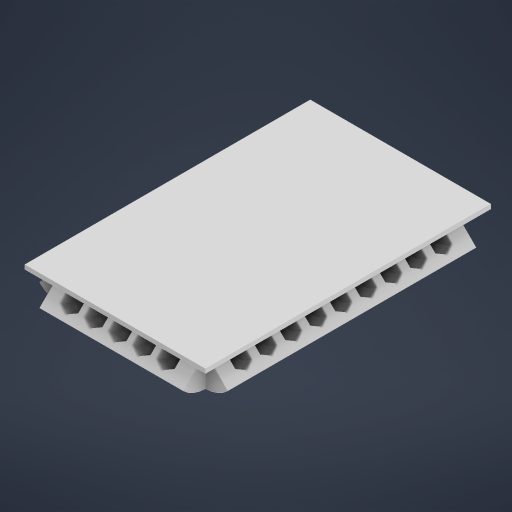
# Autodesk Inventor part: cap
Saved by Autodesk Inventor 2023 (Build 270158000, 158)
## iProperties
Created: 2022-02-14
Part Number: cap
Material: Generic
Document SubType Name: Modeling
Designer: Vlasciar
Density: 1 g/cm^3
Appearance: Default
Author: Vlasciar
Autodesk Inventor part; units mm, degrees
ref_plane "YZ Plane" through (0, 0, 0) normal (1, 0, 0) x (0, 1, 0)
ref_plane "XZ Plane" through (0, 0, 0) normal (0, 1, 0) x (-1, 0, 0)
ref_plane "XY Plane" through (0, 0, 0) normal (0, 0, 1) x (1, 0, 0)
sketch "Sketch1" plane through (0, 0, 0) normal (0, 1, 0) x (-1, 0, 0)
  line L0 (45.3593, 21.0458) -> (-32.1407, 21.0458)
  line L1 (-32.1407, 21.0458) -> (-32.1407, -112.9542)
  line L2 (-32.1407, -112.9542) -> (45.3593, -112.9542)
  line L3 (45.3593, -112.9542) -> (45.3593, 21.0458)
  line L4 (50.3593, 26.0458) -> (-37.1407, 26.0458)
  line L5 (-37.1407, 26.0458) -> (-37.1407, -117.9542)
  line L6 (-37.1407, -117.9542) -> (50.3593, -117.9542)
  line L7 (50.3593, -117.9542) -> (50.3593, 26.0458)
  point P0 (0, 0)
  dimension "d0" = 77.5
  dimension "d1" = 134
  dimension "d2" = 5
  dimension "d3" = 5
  dimension "d4" = 5
  dimension "d5" = 5
  constraints: 16 end point, 4 parallel, 2 horizontal, 2 perpendicular
  measures "d0" distance of L0.start L0.end
  measures "d1" distance of L2.end L0.start
  measures "d2" distance between parallel lines of L7 L3
  measures "d3" distance between parallel lines of L0 L4
  measures "d4" distance between parallel lines of L1 L5
  measures "d5" distance between parallel lines of L6 L2
extrude "Extrusion1" add sketch "Sketch1" against normal blind 3 contours L3 L2 L1 L0
extrude "Extrusion2" add sketch "Sketch1" along normal blind 2 contours L3 L2 L1 L0 | L7 L6 L5 L4
shell "Shell1" thickness 4 removed faces 1 at (-19.526, -3, -68.2876)
sketch "Sketch2" plane through (-41.3593, -2, 17.0458) normal (0, -1, 0) x (1, 0, 0)
  line L0 (69.5, 0) -> (69.5, -126) projected
  line L1 (0, 0) -> (69.5, 0) projected
  line L2 (0, -126) -> (0, 0) projected
  line L3 (69.5, -126) -> (0, -126) projected
  point P0 (41.3593, -17.0458)
extrude "Extrusion3" cut sketch "Sketch2" against normal blind 1
sketch "Sketch3" plane through (-41.3593, -1, 17.0458) normal (0, -1, 0) x (1, 0, 0)
  line L0 (69.5, 0) -> (69.5, -126) projected
  line L1 (0, 0) -> (69.5, 0) projected
  line L2 (60.5, -10.9282) -> (60.5, -6.3094)
  line L3 (60.5, -6.3094) -> (64.5, -4)
  line L4 (64.5, -4) -> (68.5, -6.3094)
  line L5 (68.5, -6.3094) -> (68.5, -10.9282)
  line L6 (68.5, -10.9282) -> (64.5, -13.2376)
  line L7 (64.5, -13.2376) -> (60.5, -10.9282)
  line L8 (69.5, 0) -> (69.5, -126) projected
  line L9 (0, -126) -> (0, 0) projected
  line L10 (60.5, -22.9282) -> (60.5, -18.3094)
  line L11 (60.5, -18.3094) -> (64.5, -16)
  line L12 (64.5, -16) -> (68.5, -18.3094)
  line L13 (68.5, -18.3094) -> (68.5, -22.9282)
  line L14 (68.5, -22.9282) -> (64.5, -25.2376)
  line L15 (64.5, -25.2376) -> (60.5, -22.9282)
  line L16 (60.5, -34.9282) -> (60.5, -30.3094)
  line L17 (60.5, -30.3094) -> (64.5, -28)
  line L18 (64.5, -28) -> (68.5, -30.3094)
  line L19 (68.5, -30.3094) -> (68.5, -34.9282)
  line L20 (68.5, -34.9282) -> (64.5, -37.2376)
  line L21 (64.5, -37.2376) -> (60.5, -34.9282)
  line L22 (60.5, -46.9282) -> (60.5, -42.3094)
  line L23 (60.5, -42.3094) -> (64.5, -40)
  line L24 (64.5, -40) -> (68.5, -42.3094)
  line L25 (68.5, -42.3094) -> (68.5, -46.9282)
  line L26 (68.5, -46.9282) -> (64.5, -49.2376)
  line L27 (64.5, -49.2376) -> (60.5, -46.9282)
  line L28 (60.5, -58.9282) -> (60.5, -54.3094)
  line L29 (60.5, -54.3094) -> (64.5, -52)
  line L30 (64.5, -52) -> (68.5, -54.3094)
  line L31 (68.5, -54.3094) -> (68.5, -58.9282)
  line L32 (68.5, -58.9282) -> (64.5, -61.2376)
  line L33 (64.5, -61.2376) -> (60.5, -58.9282)
  line L34 (60.5, -70.9282) -> (60.5, -66.3094)
  line L35 (60.5, -66.3094) -> (64.5, -64)
  line L36 (64.5, -64) -> (68.5, -66.3094)
  line L37 (68.5, -66.3094) -> (68.5, -70.9282)
  line L38 (68.5, -70.9282) -> (64.5, -73.2376)
  line L39 (64.5, -73.2376) -> (60.5, -70.9282)
  line L40 (60.5, -82.9282) -> (60.5, -78.3094)
  line L41 (60.5, -78.3094) -> (64.5, -76)
  line L42 (64.5, -76) -> (68.5, -78.3094)
  line L43 (68.5, -78.3094) -> (68.5, -82.9282)
  line L44 (68.5, -82.9282) -> (64.5, -85.2376)
  line L45 (64.5, -85.2376) -> (60.5, -82.9282)
  line L46 (60.5, -94.9282) -> (60.5, -90.3094)
  line L47 (60.5, -90.3094) -> (64.5, -88)
  line L48 (64.5, -88) -> (68.5, -90.3094)
  line L49 (68.5, -90.3094) -> (68.5, -94.9282)
  line L50 (68.5, -94.9282) -> (64.5, -97.2376)
  line L51 (64.5, -97.2376) -> (60.5, -94.9282)
  line L52 (60.5, -106.9282) -> (60.5, -102.3094)
  line L53 (60.5, -102.3094) -> (64.5, -100)
  line L54 (64.5, -100) -> (68.5, -102.3094)
  line L55 (68.5, -102.3094) -> (68.5, -106.9282)
  line L56 (68.5, -106.9282) -> (64.5, -109.2376)
  line L57 (64.5, -109.2376) -> (60.5, -106.9282)
  line L58 (60.5, -118.9282) -> (60.5, -114.3094)
  line L59 (60.5, -114.3094) -> (64.5, -112)
  line L60 (64.5, -112) -> (68.5, -114.3094)
  line L61 (68.5, -114.3094) -> (68.5, -118.9282)
  line L62 (68.5, -118.9282) -> (64.5, -121.2376)
  line L63 (64.5, -121.2376) -> (60.5, -118.9282)
  line L64 (48.5, -10.9282) -> (48.5, -6.3094)
  line L65 (48.5, -6.3094) -> (52.5, -4)
  line L66 (52.5, -4) -> (56.5, -6.3094)
  line L67 (56.5, -6.3094) -> (56.5, -10.9282)
  line L68 (56.5, -10.9282) -> (52.5, -13.2376)
  line L69 (52.5, -13.2376) -> (48.5, -10.9282)
  line L70 (48.5, -22.9282) -> (48.5, -18.3094)
  line L71 (48.5, -18.3094) -> (52.5, -16)
  line L72 (52.5, -16) -> (56.5, -18.3094)
  line L73 (56.5, -18.3094) -> (56.5, -22.9282)
  line L74 (56.5, -22.9282) -> (52.5, -25.2376)
  line L75 (52.5, -25.2376) -> (48.5, -22.9282)
  line L76 (48.5, -34.9282) -> (48.5, -30.3094)
  line L77 (48.5, -30.3094) -> (52.5, -28)
  line L78 (52.5, -28) -> (56.5, -30.3094)
  line L79 (56.5, -30.3094) -> (56.5, -34.9282)
  line L80 (56.5, -34.9282) -> (52.5, -37.2376)
  line L81 (52.5, -37.2376) -> (48.5, -34.9282)
  line L82 (48.5, -46.9282) -> (48.5, -42.3094)
  line L83 (48.5, -42.3094) -> (52.5, -40)
  line L84 (52.5, -40) -> (56.5, -42.3094)
  line L85 (56.5, -42.3094) -> (56.5, -46.9282)
  line L86 (56.5, -46.9282) -> (52.5, -49.2376)
  line L87 (52.5, -49.2376) -> (48.5, -46.9282)
  line L88 (48.5, -58.9282) -> (48.5, -54.3094)
  line L89 (48.5, -54.3094) -> (52.5, -52)
  line L90 (52.5, -52) -> (56.5, -54.3094)
  line L91 (56.5, -54.3094) -> (56.5, -58.9282)
  line L92 (56.5, -58.9282) -> (52.5, -61.2376)
  line L93 (52.5, -61.2376) -> (48.5, -58.9282)
  line L94 (48.5, -70.9282) -> (48.5, -66.3094)
  line L95 (48.5, -66.3094) -> (52.5, -64)
  line L96 (52.5, -64) -> (56.5, -66.3094)
  line L97 (56.5, -66.3094) -> (56.5, -70.9282)
  line L98 (56.5, -70.9282) -> (52.5, -73.2376)
  line L99 (52.5, -73.2376) -> (48.5, -70.9282)
  line L100 (48.5, -82.9282) -> (48.5, -78.3094)
  line L101 (48.5, -78.3094) -> (52.5, -76)
  line L102 (52.5, -76) -> (56.5, -78.3094)
  line L103 (56.5, -78.3094) -> (56.5, -82.9282)
  line L104 (56.5, -82.9282) -> (52.5, -85.2376)
  line L105 (52.5, -85.2376) -> (48.5, -82.9282)
  line L106 (48.5, -94.9282) -> (48.5, -90.3094)
  line L107 (48.5, -90.3094) -> (52.5, -88)
  line L108 (52.5, -88) -> (56.5, -90.3094)
  line L109 (56.5, -90.3094) -> (56.5, -94.9282)
  line L110 (56.5, -94.9282) -> (52.5, -97.2376)
  line L111 (52.5, -97.2376) -> (48.5, -94.9282)
  line L112 (48.5, -106.9282) -> (48.5, -102.3094)
  line L113 (48.5, -102.3094) -> (52.5, -100)
  line L114 (52.5, -100) -> (56.5, -102.3094)
  line L115 (56.5, -102.3094) -> (56.5, -106.9282)
  line L116 (56.5, -106.9282) -> (52.5, -109.2376)
  line L117 (52.5, -109.2376) -> (48.5, -106.9282)
  line L118 (48.5, -118.9282) -> (48.5, -114.3094)
  line L119 (48.5, -114.3094) -> (52.5, -112)
  line L120 (52.5, -112) -> (56.5, -114.3094)
  line L121 (56.5, -114.3094) -> (56.5, -118.9282)
  line L122 (56.5, -118.9282) -> (52.5, -121.2376)
  line L123 (52.5, -121.2376) -> (48.5, -118.9282)
  line L124 (36.5, -10.9282) -> (36.5, -6.3094)
  line L125 (36.5, -6.3094) -> (40.5, -4)
  line L126 (40.5, -4) -> (44.5, -6.3094)
  line L127 (44.5, -6.3094) -> (44.5, -10.9282)
  line L128 (44.5, -10.9282) -> (40.5, -13.2376)
  line L129 (40.5, -13.2376) -> (36.5, -10.9282)
  line L130 (36.5, -22.9282) -> (36.5, -18.3094)
  line L131 (36.5, -18.3094) -> (40.5, -16)
  line L132 (40.5, -16) -> (44.5, -18.3094)
  line L133 (44.5, -18.3094) -> (44.5, -22.9282)
  line L134 (44.5, -22.9282) -> (40.5, -25.2376)
  line L135 (40.5, -25.2376) -> (36.5, -22.9282)
  line L136 (36.5, -34.9282) -> (36.5, -30.3094)
  line L137 (36.5, -30.3094) -> (40.5, -28)
  line L138 (40.5, -28) -> (44.5, -30.3094)
  line L139 (44.5, -30.3094) -> (44.5, -34.9282)
  line L140 (44.5, -34.9282) -> (40.5, -37.2376)
  line L141 (40.5, -37.2376) -> (36.5, -34.9282)
  line L142 (36.5, -46.9282) -> (36.5, -42.3094)
  line L143 (36.5, -42.3094) -> (40.5, -40)
  line L144 (40.5, -40) -> (44.5, -42.3094)
  line L145 (44.5, -42.3094) -> (44.5, -46.9282)
  line L146 (44.5, -46.9282) -> (40.5, -49.2376)
  line L147 (40.5, -49.2376) -> (36.5, -46.9282)
  line L148 (36.5, -58.9282) -> (36.5, -54.3094)
  line L149 (36.5, -54.3094) -> (40.5, -52)
  line L150 (40.5, -52) -> (44.5, -54.3094)
  line L151 (44.5, -54.3094) -> (44.5, -58.9282)
  line L152 (44.5, -58.9282) -> (40.5, -61.2376)
  line L153 (40.5, -61.2376) -> (36.5, -58.9282)
  line L154 (36.5, -70.9282) -> (36.5, -66.3094)
  line L155 (36.5, -66.3094) -> (40.5, -64)
  line L156 (40.5, -64) -> (44.5, -66.3094)
  line L157 (44.5, -66.3094) -> (44.5, -70.9282)
  line L158 (44.5, -70.9282) -> (40.5, -73.2376)
  line L159 (40.5, -73.2376) -> (36.5, -70.9282)
  line L160 (36.5, -82.9282) -> (36.5, -78.3094)
  line L161 (36.5, -78.3094) -> (40.5, -76)
  line L162 (40.5, -76) -> (44.5, -78.3094)
  line L163 (44.5, -78.3094) -> (44.5, -82.9282)
  line L164 (44.5, -82.9282) -> (40.5, -85.2376)
  line L165 (40.5, -85.2376) -> (36.5, -82.9282)
  line L166 (36.5, -94.9282) -> (36.5, -90.3094)
  line L167 (36.5, -90.3094) -> (40.5, -88)
  line L168 (40.5, -88) -> (44.5, -90.3094)
  line L169 (44.5, -90.3094) -> (44.5, -94.9282)
  line L170 (44.5, -94.9282) -> (40.5, -97.2376)
  line L171 (40.5, -97.2376) -> (36.5, -94.9282)
  line L172 (36.5, -106.9282) -> (36.5, -102.3094)
  line L173 (36.5, -102.3094) -> (40.5, -100)
  line L174 (40.5, -100) -> (44.5, -102.3094)
  line L175 (44.5, -102.3094) -> (44.5, -106.9282)
  line L176 (44.5, -106.9282) -> (40.5, -109.2376)
  line L177 (40.5, -109.2376) -> (36.5, -106.9282)
  line L178 (36.5, -118.9282) -> (36.5, -114.3094)
  line L179 (36.5, -114.3094) -> (40.5, -112)
  line L180 (40.5, -112) -> (44.5, -114.3094)
  line L181 (44.5, -114.3094) -> (44.5, -118.9282)
  line L182 (44.5, -118.9282) -> (40.5, -121.2376)
  line L183 (40.5, -121.2376) -> (36.5, -118.9282)
  line L184 (24.5, -10.9282) -> (24.5, -6.3094)
  line L185 (24.5, -6.3094) -> (28.5, -4)
  line L186 (28.5, -4) -> (32.5, -6.3094)
  line L187 (32.5, -6.3094) -> (32.5, -10.9282)
  line L188 (32.5, -10.9282) -> (28.5, -13.2376)
  line L189 (28.5, -13.2376) -> (24.5, -10.9282)
  line L190 (24.5, -22.9282) -> (24.5, -18.3094)
  line L191 (24.5, -18.3094) -> (28.5, -16)
  line L192 (28.5, -16) -> (32.5, -18.3094)
  line L193 (32.5, -18.3094) -> (32.5, -22.9282)
  line L194 (32.5, -22.9282) -> (28.5, -25.2376)
  line L195 (28.5, -25.2376) -> (24.5, -22.9282)
  line L196 (24.5, -34.9282) -> (24.5, -30.3094)
  line L197 (24.5, -30.3094) -> (28.5, -28)
  line L198 (28.5, -28) -> (32.5, -30.3094)
  line L199 (32.5, -30.3094) -> (32.5, -34.9282)
  line L200 (32.5, -34.9282) -> (28.5, -37.2376)
  line L201 (28.5, -37.2376) -> (24.5, -34.9282)
  line L202 (24.5, -46.9282) -> (24.5, -42.3094)
  line L203 (24.5, -42.3094) -> (28.5, -40)
  line L204 (28.5, -40) -> (32.5, -42.3094)
  line L205 (32.5, -42.3094) -> (32.5, -46.9282)
  line L206 (32.5, -46.9282) -> (28.5, -49.2376)
  line L207 (28.5, -49.2376) -> (24.5, -46.9282)
  line L208 (24.5, -58.9282) -> (24.5, -54.3094)
  line L209 (24.5, -54.3094) -> (28.5, -52)
  line L210 (28.5, -52) -> (32.5, -54.3094)
  line L211 (32.5, -54.3094) -> (32.5, -58.9282)
  line L212 (32.5, -58.9282) -> (28.5, -61.2376)
  line L213 (28.5, -61.2376) -> (24.5, -58.9282)
  line L214 (24.5, -70.9282) -> (24.5, -66.3094)
  line L215 (24.5, -66.3094) -> (28.5, -64)
  line L216 (28.5, -64) -> (32.5, -66.3094)
  line L217 (32.5, -66.3094) -> (32.5, -70.9282)
  line L218 (32.5, -70.9282) -> (28.5, -73.2376)
  line L219 (28.5, -73.2376) -> (24.5, -70.9282)
  line L220 (24.5, -82.9282) -> (24.5, -78.3094)
  line L221 (24.5, -78.3094) -> (28.5, -76)
  line L222 (28.5, -76) -> (32.5, -78.3094)
  line L223 (32.5, -78.3094) -> (32.5, -82.9282)
  line L224 (32.5, -82.9282) -> (28.5, -85.2376)
  line L225 (28.5, -85.2376) -> (24.5, -82.9282)
  line L226 (24.5, -94.9282) -> (24.5, -90.3094)
  line L227 (24.5, -90.3094) -> (28.5, -88)
  line L228 (28.5, -88) -> (32.5, -90.3094)
  line L229 (32.5, -90.3094) -> (32.5, -94.9282)
  line L230 (32.5, -94.9282) -> (28.5, -97.2376)
  line L231 (28.5, -97.2376) -> (24.5, -94.9282)
  line L232 (24.5, -106.9282) -> (24.5, -102.3094)
  line L233 (24.5, -102.3094) -> (28.5, -100)
  line L234 (28.5, -100) -> (32.5, -102.3094)
  line L235 (32.5, -102.3094) -> (32.5, -106.9282)
  line L236 (32.5, -106.9282) -> (28.5, -109.2376)
  line L237 (28.5, -109.2376) -> (24.5, -106.9282)
  line L238 (24.5, -118.9282) -> (24.5, -114.3094)
  line L239 (24.5, -114.3094) -> (28.5, -112)
  line L240 (28.5, -112) -> (32.5, -114.3094)
  line L241 (32.5, -114.3094) -> (32.5, -118.9282)
  line L242 (32.5, -118.9282) -> (28.5, -121.2376)
  line L243 (28.5, -121.2376) -> (24.5, -118.9282)
  line L244 (12.5, -10.9282) -> (12.5, -6.3094)
  line L245 (12.5, -6.3094) -> (16.5, -4)
  line L246 (16.5, -4) -> (20.5, -6.3094)
  line L247 (20.5, -6.3094) -> (20.5, -10.9282)
  line L248 (20.5, -10.9282) -> (16.5, -13.2376)
  line L249 (16.5, -13.2376) -> (12.5, -10.9282)
  line L250 (12.5, -22.9282) -> (12.5, -18.3094)
  line L251 (12.5, -18.3094) -> (16.5, -16)
  line L252 (16.5, -16) -> (20.5, -18.3094)
  line L253 (20.5, -18.3094) -> (20.5, -22.9282)
  line L254 (20.5, -22.9282) -> (16.5, -25.2376)
  line L255 (16.5, -25.2376) -> (12.5, -22.9282)
  line L256 (12.5, -34.9282) -> (12.5, -30.3094)
  line L257 (12.5, -30.3094) -> (16.5, -28)
  line L258 (16.5, -28) -> (20.5, -30.3094)
  line L259 (20.5, -30.3094) -> (20.5, -34.9282)
  line L260 (20.5, -34.9282) -> (16.5, -37.2376)
  line L261 (16.5, -37.2376) -> (12.5, -34.9282)
  line L262 (12.5, -46.9282) -> (12.5, -42.3094)
  line L263 (12.5, -42.3094) -> (16.5, -40)
  line L264 (16.5, -40) -> (20.5, -42.3094)
  line L265 (20.5, -42.3094) -> (20.5, -46.9282)
  line L266 (20.5, -46.9282) -> (16.5, -49.2376)
  line L267 (16.5, -49.2376) -> (12.5, -46.9282)
  line L268 (12.5, -58.9282) -> (12.5, -54.3094)
  line L269 (12.5, -54.3094) -> (16.5, -52)
  line L270 (16.5, -52) -> (20.5, -54.3094)
  line L271 (20.5, -54.3094) -> (20.5, -58.9282)
  line L272 (20.5, -58.9282) -> (16.5, -61.2376)
  line L273 (16.5, -61.2376) -> (12.5, -58.9282)
  line L274 (12.5, -70.9282) -> (12.5, -66.3094)
  line L275 (12.5, -66.3094) -> (16.5, -64)
  line L276 (16.5, -64) -> (20.5, -66.3094)
  line L277 (20.5, -66.3094) -> (20.5, -70.9282)
  line L278 (20.5, -70.9282) -> (16.5, -73.2376)
  line L279 (16.5, -73.2376) -> (12.5, -70.9282)
  line L280 (12.5, -82.9282) -> (12.5, -78.3094)
  line L281 (12.5, -78.3094) -> (16.5, -76)
  line L282 (16.5, -76) -> (20.5, -78.3094)
  line L283 (20.5, -78.3094) -> (20.5, -82.9282)
  line L284 (20.5, -82.9282) -> (16.5, -85.2376)
  line L285 (16.5, -85.2376) -> (12.5, -82.9282)
  line L286 (12.5, -94.9282) -> (12.5, -90.3094)
  line L287 (12.5, -90.3094) -> (16.5, -88)
  line L288 (16.5, -88) -> (20.5, -90.3094)
  line L289 (20.5, -90.3094) -> (20.5, -94.9282)
  line L290 (20.5, -94.9282) -> (16.5, -97.2376)
  line L291 (16.5, -97.2376) -> (12.5, -94.9282)
  line L292 (12.5, -106.9282) -> (12.5, -102.3094)
  line L293 (12.5, -102.3094) -> (16.5, -100)
  line L294 (16.5, -100) -> (20.5, -102.3094)
  line L295 (20.5, -102.3094) -> (20.5, -106.9282)
  line L296 (20.5, -106.9282) -> (16.5, -109.2376)
  line L297 (16.5, -109.2376) -> (12.5, -106.9282)
  line L298 (12.5, -118.9282) -> (12.5, -114.3094)
  line L299 (12.5, -114.3094) -> (16.5, -112)
  line L300 (16.5, -112) -> (20.5, -114.3094)
  line L301 (20.5, -114.3094) -> (20.5, -118.9282)
  line L302 (20.5, -118.9282) -> (16.5, -121.2376)
  line L303 (16.5, -121.2376) -> (12.5, -118.9282)
  line L304 (0.5, -10.9282) -> (0.5, -6.3094)
  line L305 (0.5, -6.3094) -> (4.5, -4)
  line L306 (4.5, -4) -> (8.5, -6.3094)
  line L307 (8.5, -6.3094) -> (8.5, -10.9282)
  line L308 (8.5, -10.9282) -> (4.5, -13.2376)
  line L309 (4.5, -13.2376) -> (0.5, -10.9282)
  line L310 (0.5, -22.9282) -> (0.5, -18.3094)
  line L311 (0.5, -18.3094) -> (4.5, -16)
  line L312 (4.5, -16) -> (8.5, -18.3094)
  line L313 (8.5, -18.3094) -> (8.5, -22.9282)
  line L314 (8.5, -22.9282) -> (4.5, -25.2376)
  line L315 (4.5, -25.2376) -> (0.5, -22.9282)
  line L316 (0.5, -34.9282) -> (0.5, -30.3094)
  line L317 (0.5, -30.3094) -> (4.5, -28)
  line L318 (4.5, -28) -> (8.5, -30.3094)
  line L319 (8.5, -30.3094) -> (8.5, -34.9282)
  line L320 (8.5, -34.9282) -> (4.5, -37.2376)
  line L321 (4.5, -37.2376) -> (0.5, -34.9282)
  line L322 (0.5, -46.9282) -> (0.5, -42.3094)
  line L323 (0.5, -42.3094) -> (4.5, -40)
  line L324 (4.5, -40) -> (8.5, -42.3094)
  line L325 (8.5, -42.3094) -> (8.5, -46.9282)
  line L326 (8.5, -46.9282) -> (4.5, -49.2376)
  line L327 (4.5, -49.2376) -> (0.5, -46.9282)
  line L328 (0.5, -58.9282) -> (0.5, -54.3094)
  line L329 (0.5, -54.3094) -> (4.5, -52)
  line L330 (4.5, -52) -> (8.5, -54.3094)
  line L331 (8.5, -54.3094) -> (8.5, -58.9282)
  line L332 (8.5, -58.9282) -> (4.5, -61.2376)
  line L333 (4.5, -61.2376) -> (0.5, -58.9282)
  line L334 (0.5, -70.9282) -> (0.5, -66.3094)
  line L335 (0.5, -66.3094) -> (4.5, -64)
  line L336 (4.5, -64) -> (8.5, -66.3094)
  line L337 (8.5, -66.3094) -> (8.5, -70.9282)
  line L338 (8.5, -70.9282) -> (4.5, -73.2376)
  line L339 (4.5, -73.2376) -> (0.5, -70.9282)
  line L340 (0.5, -82.9282) -> (0.5, -78.3094)
  line L341 (0.5, -78.3094) -> (4.5, -76)
  line L342 (4.5, -76) -> (8.5, -78.3094)
  line L343 (8.5, -78.3094) -> (8.5, -82.9282)
  line L344 (8.5, -82.9282) -> (4.5, -85.2376)
  line L345 (4.5, -85.2376) -> (0.5, -82.9282)
  line L346 (0.5, -94.9282) -> (0.5, -90.3094)
  line L347 (0.5, -90.3094) -> (4.5, -88)
  line L348 (4.5, -88) -> (8.5, -90.3094)
  line L349 (8.5, -90.3094) -> (8.5, -94.9282)
  line L350 (8.5, -94.9282) -> (4.5, -97.2376)
  line L351 (4.5, -97.2376) -> (0.5, -94.9282)
  line L352 (0.5, -106.9282) -> (0.5, -102.3094)
  line L353 (0.5, -102.3094) -> (4.5, -100)
  line L354 (4.5, -100) -> (8.5, -102.3094)
  line L355 (8.5, -102.3094) -> (8.5, -106.9282)
  line L356 (8.5, -106.9282) -> (4.5, -109.2376)
  line L357 (4.5, -109.2376) -> (0.5, -106.9282)
  line L358 (0.5, -118.9282) -> (0.5, -114.3094)
  line L359 (0.5, -114.3094) -> (4.5, -112)
  line L360 (4.5, -112) -> (8.5, -114.3094)
  line L361 (8.5, -114.3094) -> (8.5, -118.9282)
  line L362 (8.5, -118.9282) -> (4.5, -121.2376)
  line L363 (4.5, -121.2376) -> (0.5, -118.9282)
  point P0 (41.3593, -17.0458)
  point P1 (64.5, -8.6188)
  point P2 (64.5, -20.6188)
  point P3 (64.5, -32.6188)
  point P4 (64.5, -44.6188)
  point P5 (64.5, -56.6188)
  point P6 (64.5, -68.6188)
  point P7 (64.5, -80.6188)
  point P8 (64.5, -92.6188)
  point P9 (64.5, -104.6188)
  point P10 (64.5, -116.6188)
  point P11 (52.5, -8.6188)
  point P12 (52.5, -20.6188)
  point P13 (52.5, -32.6188)
  point P14 (52.5, -44.6188)
  point P15 (52.5, -56.6188)
  point P16 (52.5, -68.6188)
  point P17 (52.5, -80.6188)
  point P18 (52.5, -92.6188)
  point P19 (52.5, -104.6188)
  point P20 (52.5, -116.6188)
  point P21 (40.5, -8.6188)
  point P22 (40.5, -20.6188)
  point P23 (40.5, -32.6188)
  point P24 (40.5, -44.6188)
  point P25 (40.5, -56.6188)
  point P26 (40.5, -68.6188)
  point P27 (40.5, -80.6188)
  point P28 (40.5, -92.6188)
  point P29 (40.5, -104.6188)
  point P30 (40.5, -116.6188)
  point P31 (28.5, -8.6188)
  point P32 (28.5, -20.6188)
  point P33 (28.5, -32.6188)
  point P34 (28.5, -44.6188)
  point P35 (28.5, -56.6188)
  point P36 (28.5, -68.6188)
  point P37 (28.5, -80.6188)
  point P38 (28.5, -92.6188)
  point P39 (28.5, -104.6188)
  point P40 (28.5, -116.6188)
  point P41 (16.5, -8.6188)
  point P42 (16.5, -20.6188)
  point P43 (16.5, -32.6188)
  point P44 (16.5, -44.6188)
  point P45 (16.5, -56.6188)
  point P46 (16.5, -68.6188)
  point P47 (16.5, -80.6188)
  point P48 (16.5, -92.6188)
  point P49 (16.5, -104.6188)
  point P50 (16.5, -116.6188)
  point P51 (4.5, -8.6188)
  point P52 (4.5, -20.6188)
  point P53 (4.5, -32.6188)
  point P54 (4.5, -44.6188)
  point P55 (4.5, -56.6188)
  point P56 (4.5, -68.6188)
  point P57 (4.5, -80.6188)
  point P58 (4.5, -92.6188)
  point P59 (4.5, -104.6188)
  point P60 (4.5, -116.6188)
  dimension "d13" = 4
  dimension "d14" = 1
  dimension "d15" = 8
  dimension "d18" = 12
  dimension "d21" = 12
  constraints: 720 end point, 2 parallel, 1 horizontal, 1 vertical, 780 other
  measures "d13" distance from line of L1 L3.end
  measures "d14" distance between parallel lines of L0 L5
  measures "d15" distance between parallel lines of L5 L2
  measures "d18" distance of point (64.5, -8.619) point (64.5, -20.619)
  measures "d21" distance of point (64.5, -8.619) point (52.5, -8.619)
extrude "Extrusion4" cut sketch "Sketch3" against normal blind 4
sketch "Sketch4" plane through (0, -3, 0) normal (0, -1, 0) x (1, 0, 0)
  line L0 (28.1407, 17.0458) -> (28.1407, -108.9542) projected
  line L1 (28.1407, -108.9542) -> (-41.3593, -108.9542) projected
  line L2 (-41.3593, -108.9542) -> (-41.3593, 17.0458) projected
  line L3 (-41.3593, 17.0458) -> (28.1407, 17.0458) projected
  line L4 (32.1407, -112.9542) -> (32.1407, 21.0458) projected
  line L5 (32.1407, 21.0458) -> (-45.3593, 21.0458) projected
  line L6 (-45.3593, 21.0458) -> (-45.3593, -112.9542) projected
  line L7 (-45.3593, -112.9542) -> (32.1407, -112.9542) projected
  point P0 (0, 0)
extrude "Extrusion5" add sketch "Sketch4" along normal blind 4
sketch "Sketch5" plane through (0, 2, 0) normal (0, 1, 0) x (1, 0, 0)
  line L0 (-50.3593, -26.0458) -> (37.1407, -26.0458) projected
  line L1 (37.1407, -26.0458) -> (37.1407, 117.9542) projected
  line L2 (37.1407, 117.9542) -> (-50.3593, 117.9542) projected
  line L3 (-50.3593, 117.9542) -> (-50.3593, -26.0458) projected
  line L4 (-50.3593, 117.9542) -> (37.1407, 117.9542)
  line L5 (37.1407, 117.9542) -> (37.1407, -26.0458)
  line L6 (37.1407, -26.0458) -> (-50.3593, -26.0458)
  line L7 (-50.3593, -26.0458) -> (-50.3593, 117.9542)
  point P0 (0, 0)
  constraints: 8 end point, 2 parallel, 1 horizontal, 1 perpendicular
extrude "Extrusion6" add sketch "Sketch5" along normal blind 0.3
sketch "Sketch6" plane through (0, -7, 0) normal (0, -1, 0) x (1, 0, 0)
  line L0 (32.1407, 21.0458) -> (-45.3593, 21.0458) projected
  line L1 (-45.3593, 21.0458) -> (-45.3593, -112.9542) projected
  line L2 (-45.3593, -112.9542) -> (32.1407, -112.9542) projected
  line L3 (32.1407, -112.9542) -> (32.1407, 21.0458) projected
  line L4 (-41.3593, -108.9542) -> (-41.3593, 17.0458) projected
  line L5 (-41.3593, 17.0458) -> (28.1407, 17.0458) projected
  line L6 (28.1407, 17.0458) -> (28.1407, -108.9542) projected
  line L7 (28.1407, -108.9542) -> (-41.3593, -108.9542) projected
  point P0 (0, 0)
extrude "Extrusion7" add sketch "Sketch6" along normal blind 10
sketch "Sketch7" plane through (0, 2.3, 0) normal (0, 1, 0) x (1, 0, 0)
  line L0 (-50.3593, -26.0458) -> (37.1407, -26.0458) projected
  line L1 (37.1407, -26.0458) -> (37.1407, 117.9542) projected
  line L2 (37.1407, 117.9542) -> (-50.3593, 117.9542) projected
  line L3 (-50.3593, 117.9542) -> (-50.3593, -26.0458) projected
  line L4 (-55.3593, -31.0458) -> (42.1407, -31.0458)
  line L5 (42.1407, -31.0458) -> (42.1407, 122.9542)
  line L6 (42.1407, 122.9542) -> (-55.3593, 122.9542)
  line L7 (-55.3593, 122.9542) -> (-55.3593, -31.0458)
  point P0 (0, 0)
  dimension "d32" = 5
  dimension "d33" = 5
  dimension "d34" = 5
  dimension "d35" = 5
  constraints: 8 end point, 2 parallel, 1 horizontal, 1 perpendicular
  measures "d32" distance between parallel lines of L5 L1
  measures "d33" distance between parallel lines of L6 L2
  measures "d34" distance between parallel lines of L7 L3
  measures "d35" distance between parallel lines of L4 L0
extrude "Extrusion8" add sketch "Sketch7" against normal blind 2.3
sketch "Sketch8" plane through (32.1407, 0, 21.0458) normal (1, 0, 0) x (0, 0, -1)
  line L0 (0, 0) -> (0, -17) projected
  line L1 (134, -17) -> (0, -17) projected
  line L2 (12.6105, -3.4548) -> (17.0654, -6.0268)
  line L3 (17.0654, -6.0268) -> (17.0654, -11.1707)
  line L4 (17.0654, -11.1707) -> (12.6105, -13.7427)
  line L5 (12.6105, -13.7427) -> (8.1557, -11.1707)
  line L6 (8.1557, -11.1707) -> (8.1557, -6.0268)
  line L7 (8.1557, -6.0268) -> (12.6105, -3.4548)
  line L8 (26.1105, -3.4548) -> (30.5654, -6.0268)
  line L9 (30.5654, -6.0268) -> (30.5654, -11.1707)
  line L10 (30.5654, -11.1707) -> (26.1105, -13.7427)
  line L11 (26.1105, -13.7427) -> (21.6557, -11.1707)
  line L12 (21.6557, -11.1707) -> (21.6557, -6.0268)
  line L13 (21.6557, -6.0268) -> (26.1105, -3.4548)
  line L14 (39.6105, -3.4548) -> (44.0654, -6.0268)
  line L15 (44.0654, -6.0268) -> (44.0654, -11.1707)
  line L16 (44.0654, -11.1707) -> (39.6105, -13.7427)
  line L17 (39.6105, -13.7427) -> (35.1557, -11.1707)
  line L18 (35.1557, -11.1707) -> (35.1557, -6.0268)
  line L19 (35.1557, -6.0268) -> (39.6105, -3.4548)
  line L20 (53.1105, -3.4548) -> (57.5654, -6.0268)
  line L21 (57.5654, -6.0268) -> (57.5654, -11.1707)
  line L22 (57.5654, -11.1707) -> (53.1105, -13.7427)
  line L23 (53.1105, -13.7427) -> (48.6557, -11.1707)
  line L24 (48.6557, -11.1707) -> (48.6557, -6.0268)
  line L25 (48.6557, -6.0268) -> (53.1105, -3.4548)
  line L26 (66.6105, -3.4548) -> (71.0654, -6.0268)
  line L27 (71.0654, -6.0268) -> (71.0654, -11.1707)
  line L28 (71.0654, -11.1707) -> (66.6105, -13.7427)
  line L29 (66.6105, -13.7427) -> (62.1557, -11.1707)
  line L30 (62.1557, -11.1707) -> (62.1557, -6.0268)
  line L31 (62.1557, -6.0268) -> (66.6105, -3.4548)
  line L32 (80.1105, -3.4548) -> (84.5654, -6.0268)
  line L33 (84.5654, -6.0268) -> (84.5654, -11.1707)
  line L34 (84.5654, -11.1707) -> (80.1105, -13.7427)
  line L35 (80.1105, -13.7427) -> (75.6557, -11.1707)
  line L36 (75.6557, -11.1707) -> (75.6557, -6.0268)
  line L37 (75.6557, -6.0268) -> (80.1105, -3.4548)
  line L38 (93.6105, -3.4548) -> (98.0654, -6.0268)
  line L39 (98.0654, -6.0268) -> (98.0654, -11.1707)
  line L40 (98.0654, -11.1707) -> (93.6105, -13.7427)
  line L41 (93.6105, -13.7427) -> (89.1557, -11.1707)
  line L42 (89.1557, -11.1707) -> (89.1557, -6.0268)
  line L43 (89.1557, -6.0268) -> (93.6105, -3.4548)
  line L44 (107.1105, -3.4548) -> (111.5654, -6.0268)
  line L45 (111.5654, -6.0268) -> (111.5654, -11.1707)
  line L46 (111.5654, -11.1707) -> (107.1105, -13.7427)
  line L47 (107.1105, -13.7427) -> (102.6557, -11.1707)
  line L48 (102.6557, -11.1707) -> (102.6557, -6.0268)
  line L49 (102.6557, -6.0268) -> (107.1105, -3.4548)
  line L50 (120.6105, -3.4548) -> (125.0654, -6.0268)
  line L51 (125.0654, -6.0268) -> (125.0654, -11.1707)
  line L52 (125.0654, -11.1707) -> (120.6105, -13.7427)
  line L53 (120.6105, -13.7427) -> (116.1557, -11.1707)
  line L54 (116.1557, -11.1707) -> (116.1557, -6.0268)
  line L55 (116.1557, -6.0268) -> (120.6105, -3.4548)
  point P0 (21.0458, 0)
  point P1 (12.6105, -8.5987)
  point P2 (26.1105, -8.5987)
  point P3 (39.6105, -8.5987)
  point P4 (53.1105, -8.5987)
  point P5 (66.6105, -8.5987)
  point P6 (80.1105, -8.5987)
  point P7 (93.6105, -8.5987)
  point P8 (107.1105, -8.5987)
  point P9 (120.6105, -8.5987)
  dimension "d40" = 13.5
  constraints: 108 end point, 1 horizontal, 1 parallel, 117 other
  measures "d40" distance of point (12.611, -8.599) point (26.111, -8.599)
extrude "Extrusion9" cut sketch "Sketch8" against normal blind 222
sketch "Sketch9" plane through (-45.3593, 0, 21.0458) normal (0, 0, 1) x (1, 0, 0)
  line L0 (0, 0) -> (77.5, 0) projected
  line L1 (0, 0) -> (0, -17) projected
  line L2 (11.9963, -2.991) -> (16.8528, -5.7949)
  line L3 (16.8528, -5.7949) -> (16.8528, -11.4026)
  line L4 (16.8528, -11.4026) -> (11.9963, -14.2065)
  line L5 (11.9963, -14.2065) -> (7.1399, -11.4026)
  line L6 (7.1399, -11.4026) -> (7.1399, -5.7949)
  line L7 (7.1399, -5.7949) -> (11.9963, -2.991)
  line L8 (24.9963, -2.991) -> (29.8528, -5.7949)
  line L9 (29.8528, -5.7949) -> (29.8528, -11.4026)
  line L10 (29.8528, -11.4026) -> (24.9963, -14.2065)
  line L11 (24.9963, -14.2065) -> (20.1399, -11.4026)
  line L12 (20.1399, -11.4026) -> (20.1399, -5.7949)
  line L13 (20.1399, -5.7949) -> (24.9963, -2.991)
  line L14 (37.9963, -2.991) -> (42.8528, -5.7949)
  line L15 (42.8528, -5.7949) -> (42.8528, -11.4026)
  line L16 (42.8528, -11.4026) -> (37.9963, -14.2065)
  line L17 (37.9963, -14.2065) -> (33.1399, -11.4026)
  line L18 (33.1399, -11.4026) -> (33.1399, -5.7949)
  line L19 (33.1399, -5.7949) -> (37.9963, -2.991)
  line L20 (50.9963, -2.991) -> (55.8528, -5.7949)
  line L21 (55.8528, -5.7949) -> (55.8528, -11.4026)
  line L22 (55.8528, -11.4026) -> (50.9963, -14.2065)
  line L23 (50.9963, -14.2065) -> (46.1399, -11.4026)
  line L24 (46.1399, -11.4026) -> (46.1399, -5.7949)
  line L25 (46.1399, -5.7949) -> (50.9963, -2.991)
  line L26 (63.9963, -2.991) -> (68.8528, -5.7949)
  line L27 (68.8528, -5.7949) -> (68.8528, -11.4026)
  line L28 (68.8528, -11.4026) -> (63.9963, -14.2065)
  line L29 (63.9963, -14.2065) -> (59.1399, -11.4026)
  line L30 (59.1399, -11.4026) -> (59.1399, -5.7949)
  line L31 (59.1399, -5.7949) -> (63.9963, -2.991)
  point P0 (45.3593, 0)
  point P1 (11.9963, -8.5987)
  point P2 (24.9963, -8.5987)
  point P3 (37.9963, -8.5987)
  point P4 (50.9963, -8.5987)
  point P5 (63.9963, -8.5987)
  dimension "d49" = 13
  constraints: 60 end point, 1 horizontal, 1 parallel, 65 other
  measures "d49" distance of point (11.996, -8.599) point (24.996, -8.599)
extrude "Extrusion10" cut sketch "Sketch9" against normal blind 222
sketch "Sketch10" plane through (32.1407, 0, 21.0458) normal (1, 0, 0) x (0, 0, -1)
  line L0 (39.6105, -13.7427) -> (35.1557, -11.1707) projected
  line L1 (35.1557, -11.1707) -> (35.1557, -6.0268) projected
  line L2 (35.1557, -6.0268) -> (39.6105, -3.4548) projected
  line L3 (39.6105, -3.4548) -> (44.0654, -6.0268) projected
  line L4 (44.0654, -6.0268) -> (44.0654, -11.1707) projected
  line L5 (44.0654, -11.1707) -> (39.6105, -13.7427) projected
  line L6 (93.6105, -13.7427) -> (89.1557, -11.1707) projected
  line L7 (89.1557, -11.1707) -> (89.1557, -6.0268) projected
  line L8 (89.1557, -6.0268) -> (93.6105, -3.4548) projected
  line L9 (93.6105, -3.4548) -> (98.0654, -6.0268) projected
  line L10 (98.0654, -6.0268) -> (98.0654, -11.1707) projected
  line L11 (98.0654, -11.1707) -> (93.6105, -13.7427) projected
  line L12 (107.1105, -13.7427) -> (102.6557, -11.1707) projected
  line L13 (102.6557, -11.1707) -> (102.6557, -6.0268) projected
  line L14 (102.6557, -6.0268) -> (107.1105, -3.4548) projected
  line L15 (107.1105, -3.4548) -> (111.5654, -6.0268) projected
  line L16 (111.5654, -6.0268) -> (111.5654, -11.1707) projected
  line L17 (111.5654, -11.1707) -> (107.1105, -13.7427) projected
  line L18 (53.1105, -13.7427) -> (48.6557, -11.1707) projected
  line L19 (48.6557, -11.1707) -> (48.6557, -6.0268) projected
  line L20 (48.6557, -6.0268) -> (53.1105, -3.4548) projected
  line L21 (53.1105, -3.4548) -> (57.5654, -6.0268) projected
  line L22 (57.5654, -6.0268) -> (57.5654, -11.1707) projected
  line L23 (57.5654, -11.1707) -> (53.1105, -13.7427) projected
  line L24 (26.1105, -13.7427) -> (21.6557, -11.1707) projected
  line L25 (21.6557, -11.1707) -> (21.6557, -6.0268) projected
  line L26 (21.6557, -6.0268) -> (26.1105, -3.4548) projected
  line L27 (26.1105, -3.4548) -> (30.5654, -6.0268) projected
  line L28 (30.5654, -6.0268) -> (30.5654, -11.1707) projected
  line L29 (30.5654, -11.1707) -> (26.1105, -13.7427) projected
  line L30 (80.1105, -13.7427) -> (75.6557, -11.1707) projected
  line L31 (75.6557, -11.1707) -> (75.6557, -6.0268) projected
  line L32 (75.6557, -6.0268) -> (80.1105, -3.4548) projected
  line L33 (80.1105, -3.4548) -> (84.5654, -6.0268) projected
  line L34 (84.5654, -6.0268) -> (84.5654, -11.1707) projected
  line L35 (84.5654, -11.1707) -> (80.1105, -13.7427) projected
  line L36 (120.6105, -13.7427) -> (116.1557, -11.1707) projected
  line L37 (116.1557, -11.1707) -> (116.1557, -6.0268) projected
  line L38 (116.1557, -6.0268) -> (120.6105, -3.4548) projected
  line L39 (120.6105, -3.4548) -> (125.0654, -6.0268) projected
  line L40 (125.0654, -6.0268) -> (125.0654, -11.1707) projected
  line L41 (125.0654, -11.1707) -> (120.6105, -13.7427) projected
  line L42 (66.6105, -13.7427) -> (62.1557, -11.1707) projected
  line L43 (62.1557, -11.1707) -> (62.1557, -6.0268) projected
  line L44 (62.1557, -6.0268) -> (66.6105, -3.4548) projected
  line L45 (66.6105, -3.4548) -> (71.0654, -6.0268) projected
  line L46 (71.0654, -6.0268) -> (71.0654, -11.1707) projected
  line L47 (71.0654, -11.1707) -> (66.6105, -13.7427) projected
  line L48 (12.6105, -13.7427) -> (8.1557, -11.1707) projected
  line L49 (8.1557, -11.1707) -> (8.1557, -6.0268) projected
  line L50 (8.1557, -6.0268) -> (12.6105, -3.4548) projected
  line L51 (12.6105, -3.4548) -> (17.0654, -6.0268) projected
  line L52 (17.0654, -6.0268) -> (17.0654, -11.1707) projected
  line L53 (17.0654, -11.1707) -> (12.6105, -13.7427) projected
  line L54 (0, 0) -> (134, 0) projected
  line L55 (0, 0) -> (0, -17) projected
  line L56 (134, -17) -> (0, -17) projected
  line L57 (134, 0) -> (134, -17) projected
  point P0 (21.0458, 0)
revolve "Revolution1" add sketch "Sketch10" angle 45 about axis through (32.1407, 0, 21.0458) along (0, 0, 1)
sketch "Sketch11" plane through (-45.3593, -17, 21.0458) normal (0, 0, 1) x (1, 0, 0)
  line L0 (37.9963, 2.7935) -> (33.1399, 5.5974) projected
  line L1 (33.1399, 5.5974) -> (33.1399, 11.2051) projected
  line L2 (33.1399, 11.2051) -> (37.9963, 14.009) projected
  line L3 (37.9963, 14.009) -> (42.8528, 11.2051) projected
  line L4 (42.8528, 11.2051) -> (42.8528, 5.5974) projected
  line L5 (42.8528, 5.5974) -> (37.9963, 2.7935) projected
  line L6 (50.9963, 2.7935) -> (46.1399, 5.5974) projected
  line L7 (46.1399, 5.5974) -> (46.1399, 11.2051) projected
  line L8 (46.1399, 11.2051) -> (50.9963, 14.009) projected
  line L9 (50.9963, 14.009) -> (55.8528, 11.2051) projected
  line L10 (55.8528, 11.2051) -> (55.8528, 5.5974) projected
  line L11 (55.8528, 5.5974) -> (50.9963, 2.7935) projected
  line L12 (24.9963, 2.7935) -> (20.1399, 5.5974) projected
  line L13 (20.1399, 5.5974) -> (20.1399, 11.2051) projected
  line L14 (20.1399, 11.2051) -> (24.9963, 14.009) projected
  line L15 (24.9963, 14.009) -> (29.8528, 11.2051) projected
  line L16 (29.8528, 11.2051) -> (29.8528, 5.5974) projected
  line L17 (29.8528, 5.5974) -> (24.9963, 2.7935) projected
  line L18 (63.9963, 2.7935) -> (59.1399, 5.5974) projected
  line L19 (59.1399, 5.5974) -> (59.1399, 11.2051) projected
  line L20 (59.1399, 11.2051) -> (63.9963, 14.009) projected
  line L21 (63.9963, 14.009) -> (68.8528, 11.2051) projected
  line L22 (68.8528, 11.2051) -> (68.8528, 5.5974) projected
  line L23 (68.8528, 5.5974) -> (63.9963, 2.7935) projected
  line L24 (11.9963, 2.7935) -> (7.1399, 5.5974) projected
  line L25 (7.1399, 5.5974) -> (7.1399, 11.2051) projected
  line L26 (7.1399, 11.2051) -> (11.9963, 14.009) projected
  line L27 (11.9963, 14.009) -> (16.8528, 11.2051) projected
  line L28 (16.8528, 11.2051) -> (16.8528, 5.5974) projected
  line L29 (16.8528, 5.5974) -> (11.9963, 2.7935) projected
  line L30 (0, 17) -> (77.5, 17) projected
  line L31 (0, 17) -> (0, 0) projected
  line L32 (77.5, 0) -> (0, 0) projected
  arc A0 (77.5, 0) -> (89.5208, 4.9792) centre (77.5, 17) ccw projected
  line L33 (77.5, 17) -> (0, 17)
  line L34 (0, 17) -> (0, 0)
  line L35 (0, 0) -> (77.5, 0)
  line L36 (77.5, 0) -> (77.5, 17)
  point P0 (45.3593, 17)
  constraints: 8 end point, 2 parallel, 1 horizontal, 1 perpendicular
sketch "Sketch12" plane through (-45.3593, 0, -112.9542) normal (-1, 0, 0) x (0, 0, 1)
  line L0 (98.8443, -11.1707) -> (94.3895, -13.7427) projected
  line L1 (94.3895, -13.7427) -> (89.9346, -11.1707) projected
  line L2 (89.9346, -11.1707) -> (89.9346, -6.0268) projected
  line L3 (89.9346, -6.0268) -> (94.3895, -3.4548) projected
  line L4 (94.3895, -3.4548) -> (98.8443, -6.0268) projected
  line L5 (98.8443, -6.0268) -> (98.8443, -11.1707) projected
  line L6 (44.8443, -11.1707) -> (40.3895, -13.7427) projected
  line L7 (40.3895, -13.7427) -> (35.9346, -11.1707) projected
  line L8 (35.9346, -11.1707) -> (35.9346, -6.0268) projected
  line L9 (35.9346, -6.0268) -> (40.3895, -3.4548) projected
  line L10 (40.3895, -3.4548) -> (44.8443, -6.0268) projected
  line L11 (44.8443, -6.0268) -> (44.8443, -11.1707) projected
  line L12 (31.3443, -11.1707) -> (26.8895, -13.7427) projected
  line L13 (26.8895, -13.7427) -> (22.4346, -11.1707) projected
  line L14 (22.4346, -11.1707) -> (22.4346, -6.0268) projected
  line L15 (22.4346, -6.0268) -> (26.8895, -3.4548) projected
  line L16 (26.8895, -3.4548) -> (31.3443, -6.0268) projected
  line L17 (31.3443, -6.0268) -> (31.3443, -11.1707) projected
  line L18 (85.3443, -11.1707) -> (80.8895, -13.7427) projected
  line L19 (80.8895, -13.7427) -> (76.4346, -11.1707) projected
  line L20 (76.4346, -11.1707) -> (76.4346, -6.0268) projected
  line L21 (76.4346, -6.0268) -> (80.8895, -3.4548) projected
  line L22 (80.8895, -3.4548) -> (85.3443, -6.0268) projected
  line L23 (85.3443, -6.0268) -> (85.3443, -11.1707) projected
  line L24 (112.3443, -11.1707) -> (107.8895, -13.7427) projected
  line L25 (107.8895, -13.7427) -> (103.4346, -11.1707) projected
  line L26 (103.4346, -11.1707) -> (103.4346, -6.0268) projected
  line L27 (103.4346, -6.0268) -> (107.8895, -3.4548) projected
  line L28 (107.8895, -3.4548) -> (112.3443, -6.0268) projected
  line L29 (112.3443, -6.0268) -> (112.3443, -11.1707) projected
  line L30 (58.3443, -11.1707) -> (53.8895, -13.7427) projected
  line L31 (53.8895, -13.7427) -> (49.4346, -11.1707) projected
  line L32 (49.4346, -11.1707) -> (49.4346, -6.0268) projected
  line L33 (49.4346, -6.0268) -> (53.8895, -3.4548) projected
  line L34 (53.8895, -3.4548) -> (58.3443, -6.0268) projected
  line L35 (58.3443, -6.0268) -> (58.3443, -11.1707) projected
  line L36 (17.8443, -11.1707) -> (13.3895, -13.7427) projected
  line L37 (13.3895, -13.7427) -> (8.9346, -11.1707) projected
  line L38 (8.9346, -11.1707) -> (8.9346, -6.0268) projected
  line L39 (8.9346, -6.0268) -> (13.3895, -3.4548) projected
  line L40 (13.3895, -3.4548) -> (17.8443, -6.0268) projected
  line L41 (17.8443, -6.0268) -> (17.8443, -11.1707) projected
  line L42 (71.8443, -11.1707) -> (67.3895, -13.7427) projected
  line L43 (67.3895, -13.7427) -> (62.9346, -11.1707) projected
  line L44 (62.9346, -11.1707) -> (62.9346, -6.0268) projected
  line L45 (62.9346, -6.0268) -> (67.3895, -3.4548) projected
  line L46 (67.3895, -3.4548) -> (71.8443, -6.0268) projected
  line L47 (71.8443, -6.0268) -> (71.8443, -11.1707) projected
  line L48 (125.8443, -11.1707) -> (121.3895, -13.7427) projected
  line L49 (121.3895, -13.7427) -> (116.9346, -11.1707) projected
  line L50 (116.9346, -11.1707) -> (116.9346, -6.0268) projected
  line L51 (116.9346, -6.0268) -> (121.3895, -3.4548) projected
  line L52 (121.3895, -3.4548) -> (125.8443, -6.0268) projected
  line L53 (125.8443, -6.0268) -> (125.8443, -11.1707) projected
  line L54 (0, 0) -> (134, 0) projected
  line L55 (0, 0) -> (0, -17) projected
  line L56 (134, -17) -> (0, -17) projected
  line L57 (134, 0) -> (134, -17) projected
  point P0 (112.9542, 0)
revolve "Revolution2" add sketch "Sketch12" angle 45 about axis through (-45.3593, 0, -112.9542) along (0, 0, -1)
revolve "Revolution3" add sketch "Sketch11" angle 45 about axis through (-45.3593, 0, 21.0458) along (-1, 0, 0)
body "Solid1"
